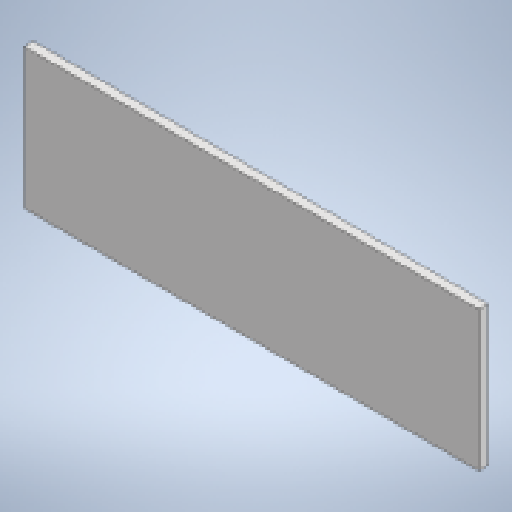
# Autodesk Inventor part: PCB_2
Saved by Autodesk Inventor 2023 (Build 270158000, 158)
## iProperties
Created: 2023-04-06
Part Number: PCB_2
Material: Ogólny
Document SubType Name: Modeling
Designer: Kamil
Density: 1 g/cm^3
Appearance: Domyślna
Author: Kamil
Autodesk Inventor part; units mm, degrees
ref_plane "YZ Plane" through (0, 0, 0) normal (1, 0, 0) x (0, 1, 0)
ref_plane "XZ Plane" through (0, 0, 0) normal (0, 1, 0) x (-1, 0, 0)
ref_plane "XY Plane" through (0, 0, 0) normal (0, 0, 1) x (1, 0, 0)
sketch "Szkic1" plane through (0, 0, 0) normal (0, 0, 1) x (1, 0, 0)
  line L0 (60.4, 41.4743) -> (60.4, -10.2735) projected
  line L1 (-23.6, 41.4743) -> (-23.6, -10.2735) projected
  arc A0 (51.3572, -8.86) -> (51.4986, -8.8014) centre (51.3572, -8.66) ccw projected
  line L2 (52.3414, -7.9586) -> (51.4986, -8.8014) projected
  arc A1 (52.4828, -7.9) -> (52.3414, -7.9586) centre (52.4828, -8.1) ccw projected
  line L3 (53.2, -7.9) -> (52.4828, -7.9) projected
  line L4 (53.2, -7.9) -> (53.2, -6.8) projected
  arc A2 (53.2, -6.8) -> (53, -6.6) centre (53, -6.8) ccw projected
  line L5 (53, -6.6) -> (48.6, -6.6) projected
  line L6 (48.6, -6.6) -> (48.6, 11.6) projected
  line L7 (48.6, 11.6) -> (25, 11.6) projected
  line L8 (25, 11.6) -> (25, -6.6) projected
  line L9 (25, -6.6) -> (20.6, -6.6) projected
  arc A3 (20.6, -6.6) -> (20.4, -6.8) centre (20.6, -6.8) ccw projected
  line L10 (20.4, -6.8) -> (20.4, -7.9) projected
  line L11 (20.4, -7.9) -> (21.0343, -7.9) projected
  arc A4 (21.3172, -8.0172) -> (21.0343, -7.9) centre (21.0343, -8.3) ccw projected
  line L12 (21.3172, -8.0172) -> (22.1014, -8.8014) projected
  arc A5 (22.1014, -8.8014) -> (22.2428, -8.86) centre (22.2428, -8.66) ccw projected
  line L13 (25, -8.86) -> (22.2428, -8.86) projected
  line L14 (25, -8.86) -> (25, -11.6) projected
  line L15 (25, -11.6) -> (28.4206, -11.6) projected
  line L16 (28.4206, -11.6) -> (28.4206, -16) projected
  line L17 (28.4206, -16) -> (32.7794, -16) projected
  line L18 (32.7794, -11.6) -> (32.7794, -16) projected
  line L19 (32.7794, -11.6) -> (48.6, -11.6) projected
  line L20 (48.6, -11.6) -> (48.6, -8.86) projected
  line L21 (48.6, -8.86) -> (51.3572, -8.86) projected
  arc A6 (-14.6986, -8.8014) -> (-14.5572, -8.86) centre (-14.5572, -8.66) ccw projected
  line L22 (-11.8, -8.86) -> (-14.5572, -8.86) projected
  line L23 (-11.8, -11.6) -> (-11.8, -8.86) projected
  line L24 (4.0206, -11.6) -> (-11.8, -11.6) projected
  line L25 (4.0206, -11.6) -> (4.0206, -16) projected
  line L26 (8.3794, -16) -> (4.0206, -16) projected
  line L27 (8.3794, -11.6) -> (8.3794, -16) projected
  line L28 (11.8, -11.6) -> (8.3794, -11.6) projected
  line L29 (11.8, -8.86) -> (11.8, -11.6) projected
  line L30 (11.8, -8.86) -> (14.5572, -8.86) projected
  arc A7 (14.5572, -8.86) -> (14.6986, -8.8014) centre (14.5572, -8.66) ccw projected
  line L31 (15.4828, -8.0172) -> (14.6986, -8.8014) projected
  arc A8 (15.7657, -7.9) -> (15.4828, -8.0172) centre (15.7657, -8.3) ccw projected
  line L32 (16.4, -7.9) -> (15.7657, -7.9) projected
  line L33 (16.4, -6.8) -> (16.4, -7.9) projected
  arc A9 (16.4, -6.8) -> (16.2, -6.6) centre (16.2, -6.8) ccw projected
  line L34 (11.8, -6.6) -> (16.2, -6.6) projected
  line L35 (11.8, 11.6) -> (11.8, -6.6) projected
  line L36 (-11.8, 11.6) -> (11.8, 11.6) projected
  line L37 (-11.8, -6.6) -> (-11.8, 11.6) projected
  line L38 (-16.2, -6.6) -> (-11.8, -6.6) projected
  arc A10 (-16.2, -6.6) -> (-16.4, -6.8) centre (-16.2, -6.8) ccw projected
  line L39 (-16.4, -7.9) -> (-16.4, -6.8) projected
  line L40 (-16.4, -7.9) -> (-15.6828, -7.9) projected
  arc A11 (-15.5414, -7.9586) -> (-15.6828, -7.9) centre (-15.6828, -8.1) ccw projected
  line L41 (-15.5414, -7.9586) -> (-14.6986, -8.8014) projected
  line L42 (60.4, 0.1) -> (-23.6, 0.1)
  line L43 (60.4, 0.1) -> (-23.6, 0.1)
  line L44 (-23.6, 0.1) -> (-23.6, 30.1)
  line L45 (-23.6, 30.1) -> (60.4, 30.1)
  line L46 (60.4, 30.1) -> (60.4, 0.1)
  line L47 (57.4, 27.1) -> (-20.6, 27.1)
  line L48 (-20.6, 27.1) -> (-20.6, 3.1)
  line L49 (-20.6, 3.1) -> (57.4, 3.1)
  line L50 (57.4, 3.1) -> (57.4, 27.1)
  point P0 (0, 0)
  dimension "d0" = 30
  dimension "d1" = 3
  constraints: 18 end point, 4 parallel, 3 point on line, 2 horizontal, 2 perpendicular, 3 other
  measures "d0" distance of L43.end L44.end
  measures "d1" distance between parallel lines of L45 L47
extrude "Wyciągnięcie proste1" add sketch "Szkic1" along normal blind 1.6 contours L49 L8 L7 L6 | L6 L7 L8 L49 L35 L36 L37 L48 L47 L50 | L37 L36 L35 L49
